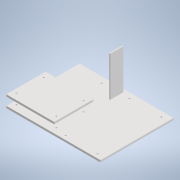
# Autodesk Inventor part: UpperChassis_Base_2
Saved by Autodesk Inventor 2020 (Build 240168000, 168)
## iProperties
Created: 2021-12-09
Part Number: UpperChassis_Base_2
Material: Generic
Document SubType Name: Modeling
Designer: danie
Density: 1 g/cm^3
Appearance: Default
Author: danie
Autodesk Inventor part; units mm, degrees
ref_plane "YZ Plane" through (0, 0, 0) normal (1, 0, 0) x (0, 1, 0)
sketch "Sketch1" plane through (0, 0, 0) normal (0, 1, 0) x (-1, 0, 0)
  line L0 (0, -0.1152) -> (-299.72, -0.1152)
  line L1 (-299.72, -0.1152) -> (-299.72, 232.9298)
  line L2 (-299.72, 232.9298) -> (0, 232.9298)
  line L3 (0, 232.9298) -> (0, -0.1152)
  line L4 (-299.72, 232.9298) -> (-293.37, 232.9298) construction
  line L5 (-293.37, 232.9298) -> (-293.37, -0.1152) construction
  line L6 (-293.37, -0.1152) -> (-299.72, -0.1152) construction
  line L7 (-299.72, -0.1152) -> (-299.72, 232.9298) construction
  line L8 (-293.37, 232.9298) -> (-290.195, 232.9298) construction
  line L9 (-290.195, 232.9298) -> (-290.195, -0.1152) construction
  line L10 (-293.37, -0.1152) -> (-293.37, 232.9298) construction
  line L11 (-290.195, 232.9298) -> (-264.795, 232.9298) construction
  line L12 (-264.795, 232.9298) -> (-264.795, 207.5298) construction
  line L13 (-264.795, 207.5298) -> (-290.195, 207.5298) construction
  line L14 (-290.195, 207.5298) -> (-290.195, 232.9298) construction
  line L15 (-264.795, 232.9298) -> (-290.195, 207.5298) construction
  line L16 (-264.795, 207.5298) -> (-290.195, 232.9298) construction
  circle A0 centre (-277.495, 220.2298) radius 2.3813
  line L17 (-264.795, 207.5298) -> (-188.595, 207.5298) construction
  line L18 (-264.795, 207.5298) -> (-188.595, 207.5298) construction
  line L19 (-188.595, 207.5298) -> (-163.195, 207.5298) construction
  line L20 (-163.195, 207.5298) -> (-163.195, 232.9298) construction
  line L21 (-163.195, 232.9298) -> (-188.595, 232.9298) construction
  line L22 (-188.595, 232.9298) -> (-188.595, 207.5298) construction
  line L23 (-163.195, 232.9298) -> (-188.595, 207.5298) construction
  line L24 (-188.595, 232.9298) -> (-163.195, 207.5298) construction
  line L25 (-290.195, -0.1152) -> (9.525, -0.1152) construction
  line L26 (9.525, -0.1152) -> (9.525, 3.1868) construction
  circle A1 centre (-175.895, 220.2298) radius 2.3813
  line L27 (-299.72, -0.1152) -> (0, -0.1152) construction
  line L28 (0, -0.1152) -> (0, 4.3298) construction
  line L29 (-299.72, 4.3298) -> (-299.72, -0.1152) construction
  line L30 (-290.195, 4.3298) -> (-264.795, 4.3298) construction
  line L31 (-264.795, 4.3298) -> (-264.795, 29.7298) construction
  line L32 (-264.795, 29.7298) -> (-290.195, 29.7298) construction
  line L33 (-290.195, 29.7298) -> (-290.195, 4.3298) construction
  line L34 (-264.795, 29.7298) -> (-188.595, 29.7298) construction
  line L35 (-188.595, 29.7298) -> (-163.195, 29.7298) construction
  line L36 (-163.195, 29.7298) -> (-163.195, 4.3298) construction
  line L37 (-163.195, 4.3298) -> (-188.595, 4.3298) construction
  line L38 (-188.595, 4.3298) -> (-188.595, 29.7298) construction
  line L39 (-163.195, 4.3298) -> (-188.595, 29.7298) construction
  line L40 (-188.595, 4.3298) -> (-163.195, 29.7298) construction
  line L41 (-264.795, 4.3298) -> (-290.195, 29.7298) construction
  line L42 (-290.195, 4.3298) -> (-264.795, 29.7298) construction
  circle A2 centre (-175.895, 17.0298) radius 2.3812
  circle A3 centre (-277.495, 17.0298) radius 2.3813
  line L43 (0, 232.9298) -> (-152.4, 232.9298) construction
  line L44 (-152.4, 232.9298) -> (-152.4, 226.5798) construction
  line L45 (-152.4, 226.5798) -> (0, 226.5798) construction
  line L46 (0, 226.5798) -> (0, 232.9298) construction
  line L47 (0, 226.5798) -> (-25.4, 226.5798) construction
  line L48 (-25.4, 226.5798) -> (-25.4, 201.1798) construction
  line L49 (-25.4, 201.1798) -> (0, 201.1798) construction
  line L50 (0, 201.1798) -> (0, 226.5798) construction
  line L51 (-152.4, 226.5798) -> (-127, 226.5798) construction
  line L52 (-127, 226.5798) -> (-127, 201.1798) construction
  line L53 (-127, 201.1798) -> (-152.4, 201.1798) construction
  line L54 (-152.4, 201.1798) -> (-152.4, 226.5798) construction
  line L55 (0, 201.1798) -> (-25.4, 226.5798) construction
  line L56 (-25.4, 201.1798) -> (0, 226.5798) construction
  line L57 (-127, 201.1798) -> (-152.4, 226.5798) construction
  line L58 (-152.4, 201.1798) -> (-127, 226.5798) construction
  circle A4 centre (-12.7, 213.8798) radius 2.3812
  circle A5 centre (-139.7, 213.8798) radius 2.3812
  line L59 (0, 226.5798) -> (-6.35, 226.5798) construction
  line L60 (-6.35, 226.5798) -> (-6.35, 114.1848) construction
  line L61 (-6.35, 114.1848) -> (0, 114.1848) construction
  line L62 (0, 114.1848) -> (0, 226.5798) construction
  line L63 (0, 114.1848) -> (-25.4, 114.1848) construction
  line L64 (-25.4, 114.1848) -> (-25.4, 139.5848) construction
  line L65 (-25.4, 139.5848) -> (0, 139.5848) construction
  line L66 (0, 139.5848) -> (0, 114.1848) construction
  line L67 (-152.4, 226.5798) -> (-146.05, 226.5798) construction
  line L68 (-146.05, 226.5798) -> (-146.05, 114.1848) construction
  line L69 (-146.05, 114.1848) -> (-152.4, 114.1848) construction
  line L70 (-152.4, 114.1848) -> (-152.4, 226.5798) construction
  line L71 (-152.4, 114.1848) -> (-127, 114.1848) construction
  line L72 (-127, 114.1848) -> (-127, 139.5848) construction
  line L73 (-127, 139.5848) -> (-152.4, 139.5848) construction
  line L74 (-152.4, 139.5848) -> (-152.4, 114.1848) construction
  line L75 (0, -0.1152) -> (-152.4, -0.1152) construction
  line L76 (-152.4, -0.1152) -> (-152.4, 6.2348) construction
  line L77 (-152.4, 6.2348) -> (0, 6.2348) construction
  line L78 (0, 6.2348) -> (0, -0.1152) construction
  line L79 (-152.4, 6.2348) -> (-127, 6.2348) construction
  line L80 (-127, 6.2348) -> (-127, 31.6348) construction
  line L81 (-127, 31.6348) -> (-152.4, 31.6348) construction
  line L82 (-152.4, 31.6348) -> (-152.4, 6.2348) construction
  line L83 (0, 114.1848) -> (-25.4, 139.5848) construction
  line L84 (-25.4, 114.1848) -> (0, 139.5848) construction
  line L85 (-127, 114.1848) -> (-152.4, 139.5848) construction
  line L86 (-152.4, 114.1848) -> (-127, 139.5848) construction
  line L87 (-127, 6.2348) -> (-152.4, 31.6348) construction
  line L88 (-152.4, 6.2348) -> (-127, 31.6348) construction
  circle A6 centre (-139.7, 18.9348) radius 2.3813
  circle A7 centre (-139.7, 126.8848) radius 2.3813
  circle A8 centre (-12.7, 126.8848) radius 2.3812
  line L89 (-152.4, -0.1152) -> (-76.2, -0.1152) construction
  line L90 (-76.2, -0.1152) -> (-76.2, 6.2348) construction
  line L91 (-76.2, 6.2348) -> (-152.4, 6.2348) construction
  line L92 (-152.4, 6.2348) -> (-152.4, -0.1152) construction
  line L93 (-76.2, 6.2348) -> (-101.6, 6.2348) construction
  line L94 (-101.6, 6.2348) -> (-101.6, 31.6348) construction
  line L95 (-101.6, 31.6348) -> (-76.2, 31.6348) construction
  line L96 (-76.2, 31.6348) -> (-76.2, 6.2348) construction
  line L97 (-76.2, 31.6348) -> (-101.6, 6.2348) construction
  line L98 (-76.2, 6.2348) -> (-101.6, 31.6348) construction
  circle A9 centre (-88.9, 18.9348) radius 2.3812
  point P0 (0, 0)
  dimension "d0" = 299.72
  dimension "d1" = 233.045
  dimension "d26" = 6.35
  dimension "d27" = 233.045
  dimension "d28" = 3.175
  dimension "d29" = 233.045
  dimension "d30" = 25.4
  dimension "d31" = 25.4
  dimension "d34" = 4.7625
  dimension "d36" = 76.2
  dimension "d38" = 25.4
  dimension "d39" = 25.4
  dimension "d44" = 3.302
  dimension "d50" = 4.7625
  dimension "d54" = 4.445
  dimension "d55" = 25.4
  dimension "d56" = 25.4
  dimension "d57" = 76.2
  dimension "d58" = 25.4
  dimension "d59" = 25.4
  dimension "d60" = 4.7625
  dimension "d61" = 4.7625
  dimension "d80" = 152.4
  dimension "d81" = 6.35
  dimension "d82" = 25.4
  dimension "d83" = 25.4
  dimension "d84" = 25.4
  dimension "d85" = 25.4
  dimension "d86" = 4.7625
  dimension "d87" = 4.7625
  dimension "d88" = 6.35
  dimension "d89" = 112.395
  dimension "d90" = 25.4
  dimension "d91" = 25.4
  dimension "d92" = 6.35
  dimension "d93" = 112.395
  dimension "d94" = 25.4
  dimension "d95" = 25.4
  dimension "d96" = 152.4
  dimension "d97" = 6.35
  dimension "d98" = 25.4
  dimension "d99" = 25.4
  dimension "d100" = 4.7625
  dimension "d101" = 4.7625
  dimension "d102" = 4.7625
  dimension "d103" = 76.2
  dimension "d104" = 6.35
  dimension "d105" = 25.4
  dimension "d106" = 25.4
  dimension "d107" = 4.7625
  constraints: 198 end point, 36 parallel, 23 horizontal, 20 perpendicular, 10 centre point, 10 midpoint, 1 collinear, 1 point on line
  measures "d0" distance of L1.end L2.end
  measures "d1" distance of L0.end L1.end
  measures "d26" distance of L5.end L6.end
  measures "d27" distance of L4.end L5.end
  measures "d28" distance of L9.end L10.start
  measures "d29" distance of L8.end L9.end
  measures "d30" distance of L12.end L13.end
  measures "d31" distance of L11.end L12.end
  measures "d34" diameter of A0
  measures "d36" distance of L12.end L17.end
  measures "d38" distance of L21.end L20.end
  measures "d39" distance of L20.end L19.end
  measures "d44" distance of L26.end L25.end
  measures "d50" diameter of A1
  measures "d54" distance of L28.end L27.end
  measures "d55" distance of L32.end L31.end
  measures "d56" distance of L31.end L30.end
  measures "d57" distance of L31.end L34.end
  measures "d58" distance of L36.end L37.end
  measures "d59" distance of L35.end L36.end
  measures "d60" diameter of A2
  measures "d61" diameter of A3
  measures "d80" distance of L45.end L44.end
  measures "d81" distance of L44.end L43.end
  measures "d82" distance of L49.end L48.end
  measures "d83" distance of L48.end L47.end
  measures "d84" distance of L52.end L53.end
  measures "d85" distance of L51.end L52.end
  measures "d86" diameter of A4
  measures "d87" diameter of A5
  measures "d88" distance of L61.end L60.end
  measures "d89" distance of L60.end L59.end
  measures "d90" distance of L64.end L65.end
  measures "d91" distance of L63.end L64.end
  measures "d92" distance of L68.end L69.end
  measures "d93" distance of L67.end L68.end
  measures "d94" distance of L73.end L72.end
  measures "d95" distance of L72.end L71.end
  measures "d96" distance of L76.end L77.end
  measures "d97" distance of L75.end L76.end
  measures "d98" distance of L81.end L80.end
  measures "d99" distance of L80.end L79.end
  measures "d100" diameter of A6
  measures "d101" diameter of A7
  measures "d102" diameter of A8
  measures "d103" distance of L91.end L90.end
  measures "d104" distance of L90.end L89.end
  measures "d105" distance of L94.end L95.end
  measures "d106" distance of L93.end L94.end
  measures "d107" diameter of A9
extrude "Extrusion1" add sketch "Sketch1" along normal blind 6.35
ref_plane "Work Plane8" through (0, 31.75, 0) normal (0, 1, 0) x (1, 0, 0)
sketch "Sketch4" plane through (0, 31.75, 0) normal (0, 1, 0) x (1, 0, 0)
  line L0 (0, -232.9298) -> (299.72, -232.9298) projected
  line L1 (0, -232.9298) -> (0, 0)
  line L2 (152.4, -232.9298) -> (0, -232.9298)
  line L3 (0, 0) -> (0, -232.9298) projected
  line L4 (76.2, -107.95) -> (0, -107.95)
  line L5 (0, -107.95) -> (0, -6.35)
  line L6 (152.4, -114.1848) -> (0, -114.1848) construction
  line L7 (152.4, -114.1848) -> (127, -114.1848) construction
  line L8 (127, -114.1848) -> (127, -139.5848) construction
  line L9 (127, -139.5848) -> (152.4, -139.5848) construction
  line L10 (152.4, -139.5848) -> (152.4, -114.1848) construction
  line L11 (0, -114.1848) -> (25.4, -114.1848) construction
  line L12 (25.4, -114.1848) -> (25.4, -139.5848) construction
  line L13 (25.4, -139.5848) -> (0, -139.5848) construction
  line L14 (0, -139.5848) -> (0, -114.1848) construction
  line L15 (0, -114.1848) -> (0, -226.5798) construction
  line L16 (0, -226.5798) -> (25.4, -226.5798) construction
  line L17 (25.4, -226.5798) -> (25.4, -201.1798) construction
  line L18 (25.4, -201.1798) -> (0, -201.1798) construction
  line L19 (0, -201.1798) -> (0, -226.5798) construction
  line L20 (152.4, -226.5798) -> (0, -226.5798) construction
  line L21 (152.4, -226.5798) -> (127, -226.5798) construction
  line L22 (127, -226.5798) -> (127, -201.1798) construction
  line L23 (127, -201.1798) -> (152.4, -201.1798) construction
  line L24 (152.4, -201.1798) -> (152.4, -226.5798) construction
  line L25 (127, -114.1848) -> (152.4, -139.5848) construction
  line L26 (152.4, -114.1848) -> (127, -139.5848) construction
  line L27 (0, -114.1848) -> (25.4, -139.5848) construction
  line L28 (0, -139.5848) -> (25.4, -114.1848) construction
  line L29 (0, -201.1798) -> (25.4, -226.5798) construction
  line L30 (25.4, -201.1798) -> (0, -226.5798) construction
  line L31 (127, -201.1798) -> (152.4, -226.5798) construction
  line L32 (152.4, -201.1798) -> (127, -226.5798) construction
  circle A0 centre (12.7, -213.8798) radius 2.3813
  circle A1 centre (139.7, -213.8798) radius 2.3813
  circle A2 centre (139.7, -126.8848) radius 2.3813
  circle A3 centre (12.7, -126.8848) radius 2.3812
  line L33 (76.2, -107.95) -> (152.4, -107.95)
  line L34 (152.4, -107.95) -> (152.4, -232.9298)
  line L35 (0, -232.9298) -> (299.72, -232.9298) projected
  point P0 (76.2, -6.35)
  point P1 (152.4, -6.35)
  dimension "d18" = 101.6
  dimension "d62" = 25.4
  dimension "d63" = 25.4
  dimension "d64" = 25.4
  dimension "d65" = 25.4
  dimension "d66" = 25.4
  dimension "d67" = 25.4
  dimension "d68" = 25.4
  dimension "d69" = 25.4
  dimension "d74" = 4.7625
  dimension "d75" = 4.7625
  dimension "d76" = 4.7625
  dimension "d77" = 4.7625
  constraints: 60 end point, 8 parallel, 8 perpendicular, 4 centre point, 4 horizontal, 4 midpoint, 1 point on line
  measures "d18" distance of point (76.2, -6.35) L4.start
  measures "d62" distance of L9.end L8.end
  measures "d63" distance of L8.end L7.end
  measures "d64" distance of L12.end L13.end
  measures "d65" distance of L11.end L12.end
  measures "d66" distance of L18.end L17.end
  measures "d67" distance of L17.end L16.end
  measures "d68" distance of L22.end L23.end
  measures "d69" distance of L21.end L22.end
  measures "d74" diameter of A0
  measures "d75" diameter of A1
  measures "d76" diameter of A2
  measures "d77" diameter of A3
extrude "Extrusion4" add sketch "Sketch4" along normal blind 6.35
ref_plane "Work Plane7" through (152.4, 6.35, 0) normal (0, 0, -1) x (-1, 0, 0)
sketch "Sketch6" plane through (152.4, 6.35, 0) normal (0, 0, -1) x (-1, 0, 0)
  line L0 (152.4, 54.61) -> (0, 54.61) construction
  line L1 (0, 48.26) -> (152.4, 48.26) construction
  line L2 (76.2, 54.61) -> (0, 54.61) construction
  line L3 (0, 54.61) -> (0, 48.26) construction
  line L4 (0, 48.26) -> (76.2, 48.26) construction
  line L5 (76.2, 48.26) -> (76.2, 54.61) construction
  line L6 (0, 48.26) -> (25.4, 48.26) construction
  line L7 (25.4, 48.26) -> (25.4, 24.13) construction
  line L8 (25.4, 24.13) -> (0, 24.13) construction
  line L9 (0, 24.13) -> (0, 48.26) construction
  line L10 (25.4, 24.13) -> (0, 48.26) construction
  line L11 (0, 24.13) -> (25.4, 48.26) construction
  line L12 (0, 0) -> (-147.32, 0) construction
  line L13 (25.4, 24.13) -> (0, 0) construction
  line L14 (0, 0) -> (25.4, 0) construction
  line L15 (0, 0) -> (25.4, 0) construction
  line L16 (25.4, 0) -> (0, 24.13) construction
  line L17 (76.2, 48.26) -> (50.8, 48.26) construction
  line L18 (50.8, 48.26) -> (50.8, 24.13) construction
  line L19 (50.8, 24.13) -> (76.2, 24.13) construction
  line L20 (76.2, 24.13) -> (76.2, 48.26) construction
  line L21 (-147.32, 0) -> (152.4, 0) construction
  line L22 (50.8, 24.13) -> (76.2, 24.13) construction
  line L23 (76.2, 24.13) -> (76.2, 0) construction
  line L24 (76.2, 0) -> (50.8, 0) construction
  line L25 (50.8, 0) -> (50.8, 24.13) construction
  line L26 (50.8, 48.26) -> (76.2, 24.13) construction
  line L27 (76.2, 0) -> (76.2, 48.26) construction
  line L28 (76.2, 48.26) -> (50.8, 24.13) construction
  line L29 (50.8, 24.13) -> (76.2, 0) construction
  line L30 (76.2, 24.13) -> (50.8, 0) construction
  circle A0 centre (12.7, 36.195) radius 2.3812
  circle A1 centre (63.5, 36.195) radius 2.3812
  circle A2 centre (63.5, 12.065) radius 2.3812
  circle A3 centre (12.7, 12.065) radius 2.3813
  point P0 (152.4, -6.35)
  dimension "d108" = 76.2
  dimension "d109" = 6.35
  dimension "d110" = 25.4
  dimension "d111" = 24.13
  dimension "d112" = 25.4
  dimension "d114" = 25.4
  dimension "d115" = 24.13
  dimension "d116" = 4.7625
  dimension "d117" = 4.7625
  dimension "d118" = 4.7625
  dimension "d119" = 4.7625
  constraints: 52 end point, 8 parallel, 6 horizontal, 5 midpoint, 4 centre point, 4 perpendicular, 2 point on line, 1 collinear
  measures "d108" distance of L4.end L1.start
  measures "d109" distance of L1.start L2.end
  measures "d110" distance of L7.end L8.end
  measures "d111" distance of L6.end L7.end
  measures "d112" distance of L12.start L14.end
  measures "d114" distance of L19.end L18.end
  measures "d115" distance of L18.end L17.end
  measures "d116" diameter of A0
  measures "d117" diameter of A1
  measures "d118" diameter of A2
  measures "d119" diameter of A3
extrude "Extrusion5" cut sketch "Sketch6" against normal blind 6.35
sketch "Sketch11" plane through (0, 6.35, 0) normal (0, 1, 0) x (1, 0, 0)
  line L0 (145.5925, -51.0146) -> (148.7675, -51.0146)
  line L1 (148.7675, -51.0146) -> (148.7675, -9.4234)
  line L2 (148.7675, -9.4234) -> (145.5925, -9.4234)
  line L3 (145.5925, -9.4234) -> (145.5925, -51.0146)
  point P0 (0, 0)
  dimension "d169" = 3.175
  constraints: 8 end point, 2 parallel, 1 horizontal, 1 perpendicular
  measures "d169" distance of L2.end L1.end
extrude "Extrusion8" add sketch "Sketch11" along normal blind 127
body "Solid1"
